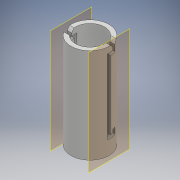
# Autodesk Inventor part: RescueKitThrow_pipe
Saved by Autodesk Inventor 2018.3 (Build 223284000, 284)
## iProperties
Created: 2019-02-10
Part Number: RescueKitThrow_pipe
Material: 一般
Document SubType Name: Modeling
Designer: shun2
Density: 1 g/cm^3
Appearance: 既定
Author: shun2
Autodesk Inventor part; units mm, degrees
ref_plane "XZ Plane" through (0, 0, 0) normal (0, 1, 0) x (-1, 0, 0)
ref_plane "XY Plane" through (0, 0, 0) normal (0, 0, 1) x (1, 0, 0)
sketch "スケッチ1" plane through (0, 0, 0) normal (0, 0, 1) x (1, 0, 0)
  circle A0 centre (0, 0) radius 13
  circle A1 centre (0, 0) radius 0.6
  dimension "d0" = 26
  dimension "d1" = 1.2
  constraints: 2 centre point, 2 coincident
  measures "d0" diameter of A0
  measures "d1" diameter of A1
extrude "押し出し1" add sketch "スケッチ1" along normal blind 5
sketch "スケッチ2" plane through (0, 0, 5) normal (0, 0, 1) x (1, 0, 0)
  circle A0 centre (0, 0) radius 13
  circle A1 centre (0, 0) radius 0.6 projected
  circle A2 centre (0, 0) radius 10
  dimension "d4" = 26
  dimension "d5" = 20
  constraints: 2 centre point, 2 coincident
  measures "d4" diameter of A0
  measures "d5" diameter of A2
extrude "押し出し2" add sketch "スケッチ2" along normal blind 60 contours A0
ref_plane "作業平面1" through (13, 0, 0) normal (1, 0, 0) x (0, 1, 0)
sketch "スケッチ3" plane through (13, 0, 0) normal (1, 0, 0) x (0, 1, 0)
  line L0 (-13, 0) -> (13, 0) projected
  line L1 (-13, 0) -> (-13, 65) projected
  line L2 (13, 0) -> (13, 65) projected
  line L3 (-1, 59) -> (1, 59)
  line L4 (1, 59) -> (1, 10)
  line L5 (1, 10) -> (-1, 10)
  line L6 (-1, 10) -> (-1, 59)
  point P0 (0, 0)
  dimension "d27" = 2
  dimension "d28" = 49
  constraints: 8 end point, 2 parallel, 1 horizontal, 1 perpendicular
  measures "d27" distance of L4.end L5.end
  measures "d28" distance of L3.end L4.end
extrude "押し出し3" cut sketch "スケッチ3" against normal blind 30
sketch "スケッチ4" plane through (13, 0, 0) normal (1, 0, 0) x (0, 1, 0)
  line L0 (1, 10) -> (-1, 10) projected
  line L1 (-1, 10) -> (5, 10)
  line L2 (5, 10) -> (5, 12)
  line L3 (3, 12) -> (-1, 12)
  line L4 (-1, 12) -> (-1, 10)
  line L5 (5, 10) -> (3, 10)
  line L6 (3, 12) -> (3, 14)
  line L7 (3, 14) -> (5, 14)
  line L8 (5, 14) -> (5, 10)
  line L9 (-1, 10) -> (-1, 59) projected
  line L10 (-1, 59) -> (5, 59)
  line L11 (5, 59) -> (5, 61)
  line L12 (3, 61) -> (-1, 61)
  line L13 (-1, 61) -> (-1, 59)
  line L14 (5, 59) -> (3, 59)
  line L15 (3, 61) -> (3, 65)
  line L16 (3, 65) -> (5, 65)
  line L17 (5, 65) -> (5, 59)
  point P0 (0, 0)
  dimension "d12" = 6
  dimension "d13" = 2
  dimension "d14" = 2
  dimension "d15" = 4
  dimension "d33" = 6
  dimension "d34" = 2
  dimension "d35" = 6
  constraints: 32 end point, 8 parallel, 4 horizontal, 4 perpendicular
  measures "d12" distance of L3.end L2.end
  measures "d13" distance of L2.end L1.end
  measures "d14" distance of L6.end L7.end
  measures "d15" distance of L5.end L6.end
  measures "d33" distance of L12.end L11.end
  measures "d34" distance of L11.end L10.end
  measures "d35" distance of L14.end L15.end
extrude "押し出し4" cut sketch "スケッチ4" against normal blind 8
ref_plane "作業平面2" through (-13, 0, 0) normal (1, 0, 0) x (0, 1, 0)
sketch "スケッチ5" plane through (-13, 0, 0) normal (1, 0, 0) x (0, 1, 0)
  line L0 (5, 10) -> (-1, 10) projected
  line L1 (1, 10) -> (-5, 10)
  line L2 (-5, 10) -> (-5, 12)
  line L3 (-3, 12) -> (1, 12)
  line L4 (1, 12) -> (1, 10)
  line L5 (-5, 10) -> (-3, 10)
  line L6 (-3, 12) -> (-3, 14)
  line L7 (-3, 14) -> (-5, 14)
  line L8 (-5, 14) -> (-5, 10)
  line L9 (-1, 59) -> (1, 59) projected
  line L10 (1, 59) -> (-5, 59)
  line L11 (-5, 59) -> (-5, 61)
  line L12 (-3, 61) -> (1, 61)
  line L13 (1, 61) -> (1, 59)
  line L14 (-5, 59) -> (-3, 59)
  line L15 (-3, 61) -> (-3, 65)
  line L16 (-3, 65) -> (-5, 65)
  line L17 (-5, 65) -> (-5, 59)
  point P0 (0, 0)
  dimension "d18" = 6
  dimension "d19" = 2
  dimension "d20" = 2
  dimension "d21" = 4
  dimension "d29" = 6
  dimension "d30" = 2
  dimension "d31" = 2
  dimension "d32" = 6
  constraints: 32 end point, 8 parallel, 4 horizontal, 4 perpendicular, 1 point on line
  measures "d18" distance of L2.end L3.end
  measures "d19" distance of L1.end L2.end
  measures "d20" distance of L7.end L6.end
  measures "d21" distance of L6.end L5.end
  measures "d29" distance of L11.end L12.end
  measures "d30" distance of L10.end L11.end
  measures "d31" distance of L16.end L15.end
  measures "d32" distance of L15.end L14.end
extrude "押し出し5" cut sketch "スケッチ5" along normal blind 8
chamfer "面取り2" distance 2 angle 45 4 edges at (-11.0943, -3, 65) (-10.3301, -5, 65) (11.0943, 3, 65) (10.3301, 5, 65)
